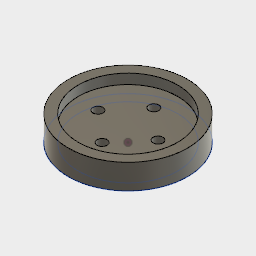
fastener (Autodesk Fusion 360 design; units mm, degrees)
Autodesk Fusion 360 part; units mm, degrees
sketch "草图1" plane through (0, 0, 0) normal (0, 1, 0) x (1, 0, 0)
  circle A0 centre (0, 0) radius 10
  circle A1 centre (0, 0) radius 12
  dimension "d1" = 2
extrude "拉伸1" add sketch "草图1" along normal blind 3 contours A0 makes body 1
extrude "拉伸2" add sketch "草图1" along normal blind 5 separate body makes body 2
cylinder "圆柱体基本要素1" add diameter 2 height 20 placed x (1, 0, 0) y (0, 1, 0) z (0, 0, 1) at (25, 6, 0) separate body makes body 3
move_body "对齐1" bodies 3 to x (1, 0, 0) y (0, 0, -1) z (0, 1, 0) at (0, -17, 26)
move_body "对齐2" bodies 3 to x (1, 0, 0) y (0, 1, 0) z (0, 0, 1) at (0, 0, 0)
move_face "MoveFace1" to x (1, 0, 0) y (0, 1, 0) z (0, 0, 1) at (-32.3377, 51.9185, -19.5808) 1 faces at (25.7971, -10.3333, 19.3962) on bodies 3
move_face "MoveFace2" to x (1, 0, 0) y (0, 1, 0) z (0, 0, 1) at (1.71, -0.1026, 0) 1 faces at (-6.3426, -3.6667, 0.5188) on bodies 3
move_face "偏移面1" offset 3 1 faces at (-4.9861, 3, 0.6905) on bodies 3
pattern_circular "C-阵列1" count 4 over 360 about axis through (0, 1.75, 0) along (0, 1, 0) of bodies 3 makes body 4 at (0.5188, -1.6667, 4.6326) makes body 5 at (4.6326, -1.6667, -0.5188) makes body 6 at (-0.5188, -1.6667, -4.6326)
combine "合并1" operation cut target body 1 tool bodies 5 6 3 4
